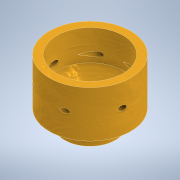
# Autodesk Inventor part: bottom injector
Saved by Autodesk Inventor 2021 (Build 250183000, 183)
## iProperties
Created: 2021-07-21
Part Number: bottom injector
Material: Brass, Soft Yellow, Welded
Document SubType Name: Modeling
Designer: samlo
Density: 8.5 g/cm^3
Appearance: Weld - Brass
Author: samlo
Autodesk Inventor part; units mm, degrees
ref_plane "YZ Plane" through (0, 0, 0) normal (1, 0, 0) x (0, 1, 0)
ref_plane "XZ Plane" through (0, 0, 0) normal (0, 1, 0) x (-1, 0, 0)
sketch "Sketch1" plane through (0, 0, 0) normal (0, 0, 1) x (1, 0, 0)
  line L0 (4, 0) -> (4, 3)
  line L1 (4, 3) -> (6.5, 6.1225)
  line L2 (6.5, 6.1225) -> (6.5, 12.1225)
  line L3 (6.5, 12.1225) -> (8, 12.1225)
  line L4 (8, 12.1225) -> (8, 3)
  line L5 (8, 3) -> (5, 3)
  line L6 (5, 3) -> (5, 0)
  line L7 (5, 0) -> (4, 0)
  line L8 (0, -2.6844) -> (0, 16.1063) projected
  point P0 (0, 0)
  dimension "d0" = 6.5
  dimension "d2" = 1.5
  dimension "d7" = 3
  dimension "d31" = 4
  dimension "d32" = 1
  dimension "d33" = 0
  dimension "d35" = 3
  dimension "d36" = 6
  dimension "d37" = 4
  constraints: 16 end point, 5 perpendicular, 1 parallel, 1 vertical
  measures "d0" distance from line of L2 point (0, 0)
  measures "d2" distance of L2.end L3.end
  measures "d7" distance of L0.start L0.end
  measures "d31" distance of L0.start point (0, 0)
  measures "d32" distance of L6.end L0.start
  measures "d33" vertical distance of L0.start point (0, 0)
  measures "d35" distance of L5.end L6.end
  measures "d36" distance of L1.end L2.end
  measures "d37" distance of L0.end L1.end
revolve "Revolution1" add sketch "Sketch1" angle 360 about axis through (0, -10, 0) along (0, 1, 0)
sketch "Sketch2" plane through (0, 0, 0) normal (1, 0, 0) x (0, 1, 0)
  line L0 (6.1225, 6.5) -> (12.1225, 6.5) projected
  point P0 (0, 0)
  point P1 (13.4219, 6.5)
  constraints: 1 point on line
ref_plane "Work Plane1" through (0, 13.4219, 6.5) normal (0, 0, -1) x (-1, 0, 0)
sketch "Sketch4" plane through (0, 0, 0) normal (1, 0, 0) x (0, 1, 0)
  line L0 (6.1225, 6.5) -> (6.1225, -6.5) projected
  line L1 (16.1063, 6.5) -> (-2.6844, 6.5) projected
  point P0 (0, 0)
  point P1 (7.6225, 6)
  dimension "d19" = 1.5
  dimension "d20" = 0.5
  measures "d19" distance from line of L0 point (7.622, 6)
  measures "d20" distance from line of L1 point (7.622, 6)
hole "Hole2" at (0, 7.6225, 6) direction (-1, 0, 0) diameter 1 end through all
pattern_circular "Circular Pattern1" count 6 over 360 about axis through (0, -10, 0) along (0, 1, 0) of "Hole2"
body "Solid1"
